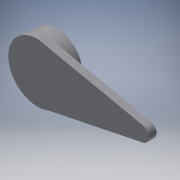
# Autodesk Inventor part: sERVOsHAFKkEY
Saved by Autodesk Inventor 2017 (Build 210142000, 142)
## iProperties
Created: 2020-08-23
Part Number: sERVOsHAFKkEY
Material: Generic
Document SubType Name: Modeling
Designer: agustin
Density: 1 g/cm^3
Appearance: Default
Author: agustin
Autodesk Inventor part; units mm, degrees
ref_plane "YZ Plane" through (0, 0, 0) normal (1, 0, 0) x (0, 1, 0)
ref_plane "XZ Plane" through (0, 0, 0) normal (0, 1, 0) x (-1, 0, 0)
ref_plane "XY Plane" through (0, 0, 0) normal (0, 0, 1) x (1, 0, 0)
sketch "Sketch1" plane through (0, 0, 0) normal (0, 0, 1) x (1, 0, 0)
  circle A0 centre (0, -0.8499) radius 4.5
  circle A1 centre (0, -0.8499) radius 6.8
  ellipse E0 centre (-17.0343, 4.4205) end of major axis (-13.1075, 2.2226) minor radius 4.4388 projected
  point P0 (0, 0)
  dimension "d0" = 13.6
  constraints: 2 centre point, 1 coincident, 2 other
  measures "d0" diameter of A1
extrude "Extrusion1" add sketch "Sketch1" along normal blind 6 contours A0 | A1
sketch "Sketch2" plane through (0, -0.8499, 6) normal (0, 0, 1) x (1, 0, 0)
  arc A0 (1.0461, 7.7621) -> (3.927, -7.1445) centre (0.9506, 0.012) ccw
  circle A1 centre (0, 0) radius 6.8 projected
  line L0 (28.8097, -2.0169) -> (3.927, -7.1445)
  line L1 (1.0461, 7.7621) -> (28.8191, 1.8988)
  arc A2 (28.8097, -2.0169) -> (28.8191, 1.8988) centre (28.406, -0.058) ccw
  point P0 (0, 0.8499)
  dimension "d4" = 2
  constraints: 4 end point, 4 point on circle, 2 centre point, 2 tangent
  measures "d4" radius of A2
extrude "Extrusion2" add sketch "Sketch2" against normal blind 2 contours A1 | L1 A2 L0 A0
scale "Scale1" factors (0.5, 0.5, 0.5) then translate (0.4753, -0.419, 3) bodies 1
body "Solid1"
